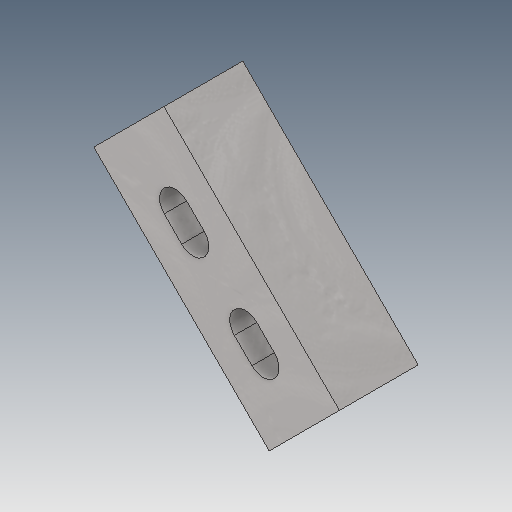
# Autodesk Inventor part: Conduit-brace
Saved by Autodesk Inventor 2017 (Build 210142000, 142)
## iProperties
Created: 2018-08-09
Part Number: Conduit-brace
Material: Generic
Document SubType Name: Modeling
Designer: Kathryn Rosie
Density: 1 g/cm^3
Appearance: Weld - Steel Mild
Author: Kathryn Rosie
Autodesk Inventor part; units mm, degrees
ref_plane "YZ Plane" through (0, 0, 0) normal (1, 0, 0) x (0, 1, 0)
ref_plane "XZ Plane" through (0, 0, 0) normal (0, 1, 0) x (-1, 0, 0)
ref_plane "XY Plane" through (0, 0, 0) normal (0, 0, 1) x (1, 0, 0)
sketch "Sketch1" plane through (0, 0, 0) normal (0, 0, 1) x (1, 0, 0)
  line L0 (7.0711, 21.2132) -> (20.3934, 34.5355)
  line L1 (61, 1) -> (41.6066, 20.3934)
  line L2 (61, 1) -> (725, 1)
  line L3 (725, 1) -> (725, 26)
  line L4 (725, 26) -> (720, 31)
  line L5 (720, 31) -> (437.7615, 31)
  arc A0 (434.226, 32.4645) -> (437.7615, 31) centre (437.7615, 36) ccw
  line L6 (434.226, 32.4645) -> (32.4645, 434.226)
  arc A1 (31, 437.7615) -> (32.4645, 434.226) centre (36, 437.7615) ccw
  line L7 (31, 437.7615) -> (31, 720)
  line L8 (31, 720) -> (26, 725)
  line L9 (26, 725) -> (1, 725)
  line L10 (1, 725) -> (1, 61)
  line L11 (20.3934, 41.6066) -> (1, 61)
  arc A2 (20.3934, 34.5355) -> (20.3934, 41.6066) centre (16.8579, 38.0711) ccw
  line L12 (7.0711, 21.2132) -> (20.3934, 34.5355)
  line L13 (21.2132, 7.0711) -> (7.0711, 21.2132)
  line L14 (34.5355, 20.3934) -> (21.2132, 7.0711)
  arc A3 (41.6066, 20.3934) -> (34.5355, 20.3934) centre (38.0711, 16.8579) ccw
  circle A4 centre (15, 600) radius 3.2
  circle A5 centre (200, 15) radius 3.2
  circle A6 centre (600, 15) radius 3.2
  line L15 (252.9319, 164.2611) -> (377.6575, 39.5355)
  arc A7 (374.1219, 31) -> (377.6575, 39.5355) centre (374.1219, 36) ccw
  line L16 (374.1219, 31) -> (82.5685, 31)
  arc A8 (79.033, 32.4645) -> (82.5685, 31) centre (82.5685, 36) ccw
  line L17 (79.033, 32.4645) -> (32.4645, 79.033)
  arc A9 (31, 82.5685) -> (32.4645, 79.033) centre (36, 82.5685) ccw
  line L18 (31, 82.5685) -> (31, 374.1219)
  arc A10 (39.5355, 377.6575) -> (31, 374.1219) centre (36, 374.1219) ccw
  line L19 (39.5355, 377.6575) -> (164.2611, 252.9319)
  arc A11 (162.7002, 244.8028) -> (164.2611, 252.9319) centre (160.7256, 249.3963) ccw
  arc A12 (162.7002, 244.8028) -> (244.8028, 162.7002) centre (187.3833, 187.3833) ccw
  arc A13 (252.9319, 164.2611) -> (244.8028, 162.7002) centre (249.3963, 160.7256) ccw
  circle A14 centre (15, 200) radius 3.2
  line L20 (-61, -1) -> (-41.6066, -20.3934)
  line L21 (-61, -1) -> (-725, -1)
  line L22 (-725, -1) -> (-725, -26)
  line L23 (-725, -26) -> (-720, -31)
  line L24 (-720, -31) -> (-437.7615, -31)
  arc A15 (-434.226, -32.4645) -> (-437.7615, -31) centre (-437.7615, -36) ccw
  line L25 (-434.226, -32.4645) -> (-32.4645, -434.226)
  arc A16 (-31, -437.7615) -> (-32.4645, -434.226) centre (-36, -437.7615) ccw
  line L26 (-31, -437.7615) -> (-31, -720)
  line L27 (-31, -720) -> (-26, -725)
  line L28 (-26, -725) -> (-1, -725)
  line L29 (-1, -725) -> (-1, -61)
  line L30 (-20.3934, -41.6066) -> (-1, -61)
  arc A17 (-20.3934, -34.5355) -> (-20.3934, -41.6066) centre (-16.8579, -38.0711) ccw
  line L31 (-7.0711, -21.2132) -> (-20.3934, -34.5355)
  line L32 (-21.2132, -7.0711) -> (-7.0711, -21.2132)
  line L33 (-34.5355, -20.3934) -> (-21.2132, -7.0711)
  arc A18 (-41.6066, -20.3934) -> (-34.5355, -20.3934) centre (-38.0711, -16.8579) ccw
  circle A19 centre (-15, -600) radius 3.2
  circle A20 centre (-200, -15) radius 3.2
  circle A21 centre (-600, -15) radius 3.2
  line L34 (-252.9319, -164.2611) -> (-377.6575, -39.5355)
  arc A22 (-374.1219, -31) -> (-377.6575, -39.5355) centre (-374.1219, -36) ccw
  line L35 (-374.1219, -31) -> (-82.5685, -31)
  arc A23 (-79.033, -32.4645) -> (-82.5685, -31) centre (-82.5685, -36) ccw
  line L36 (-79.033, -32.4645) -> (-32.4645, -79.033)
  arc A24 (-31, -82.5685) -> (-32.4645, -79.033) centre (-36, -82.5685) ccw
  line L37 (-31, -82.5685) -> (-31, -374.1219)
  arc A25 (-39.5355, -377.6575) -> (-31, -374.1219) centre (-36, -374.1219) ccw
  line L38 (-39.5355, -377.6575) -> (-164.2611, -252.9319)
  arc A26 (-162.7002, -244.8028) -> (-164.2611, -252.9319) centre (-160.7256, -249.3963) ccw
  arc A27 (-162.7002, -244.8028) -> (-244.8028, -162.7002) centre (-187.3833, -187.3833) ccw
  arc A28 (-252.9319, -164.2611) -> (-244.8028, -162.7002) centre (-249.3963, -160.7256) ccw
  circle A29 centre (-15, -200) radius 3.2
  line L39 (-1, 61) -> (-20.3934, 41.6066)
  line L40 (-1, 61) -> (-1, 725)
  line L41 (-1, 725) -> (-26, 725)
  line L42 (-26, 725) -> (-31, 720)
  line L43 (-31, 720) -> (-31, 437.7615)
  arc A30 (-32.4645, 434.226) -> (-31, 437.7615) centre (-36, 437.7615) ccw
  line L44 (-32.4645, 434.226) -> (-434.226, 32.4645)
  arc A31 (-437.7615, 31) -> (-434.226, 32.4645) centre (-437.7615, 36) ccw
  line L45 (-437.7615, 31) -> (-720, 31)
  line L46 (-720, 31) -> (-725, 26)
  line L47 (-725, 26) -> (-725, 1)
  line L48 (-725, 1) -> (-61, 1)
  line L49 (-41.6066, 20.3934) -> (-61, 1)
  arc A32 (-34.5355, 20.3934) -> (-41.6066, 20.3934) centre (-38.0711, 16.8579) ccw
  line L50 (-21.2132, 7.0711) -> (-34.5355, 20.3934)
  line L51 (-7.0711, 21.2132) -> (-21.2132, 7.0711)
  line L52 (-20.3934, 34.5355) -> (-7.0711, 21.2132)
  arc A33 (-20.3934, 41.6066) -> (-20.3934, 34.5355) centre (-16.8579, 38.0711) ccw
  circle A34 centre (-600, 15) radius 3.2
  circle A35 centre (-15, 200) radius 3.2
  circle A36 centre (-15, 600) radius 3.2
  line L53 (-164.2611, 252.9319) -> (-39.5355, 377.6575)
  arc A37 (-31, 374.1219) -> (-39.5355, 377.6575) centre (-36, 374.1219) ccw
  line L54 (-31, 374.1219) -> (-31, 82.5685)
  arc A38 (-32.4645, 79.033) -> (-31, 82.5685) centre (-36, 82.5685) ccw
  line L55 (-32.4645, 79.033) -> (-79.033, 32.4645)
  arc A39 (-82.5685, 31) -> (-79.033, 32.4645) centre (-82.5685, 36) ccw
  line L56 (-82.5685, 31) -> (-374.1219, 31)
  arc A40 (-377.6575, 39.5355) -> (-374.1219, 31) centre (-374.1219, 36) ccw
  line L57 (-377.6575, 39.5355) -> (-252.9319, 164.2611)
  arc A41 (-244.8028, 162.7002) -> (-252.9319, 164.2611) centre (-249.3963, 160.7256) ccw
  arc A42 (-244.8028, 162.7002) -> (-162.7002, 244.8028) centre (-187.3833, 187.3833) ccw
  arc A43 (-164.2611, 252.9319) -> (-162.7002, 244.8028) centre (-160.7256, 249.3963) ccw
  circle A44 centre (-200, 15) radius 3.2
  line L58 (1, -61) -> (20.3934, -41.6066)
  line L59 (1, -61) -> (1, -725)
  line L60 (1, -725) -> (26, -725)
  line L61 (26, -725) -> (31, -720)
  line L62 (31, -720) -> (31, -437.7615)
  arc A45 (32.4645, -434.226) -> (31, -437.7615) centre (36, -437.7615) ccw
  line L63 (32.4645, -434.226) -> (434.226, -32.4645)
  arc A46 (437.7615, -31) -> (434.226, -32.4645) centre (437.7615, -36) ccw
  line L64 (437.7615, -31) -> (720, -31)
  line L65 (720, -31) -> (725, -26)
  line L66 (725, -26) -> (725, -1)
  line L67 (725, -1) -> (61, -1)
  line L68 (41.6066, -20.3934) -> (61, -1)
  arc A47 (34.5355, -20.3934) -> (41.6066, -20.3934) centre (38.0711, -16.8579) ccw
  line L69 (21.2132, -7.0711) -> (34.5355, -20.3934)
  line L70 (7.0711, -21.2132) -> (21.2132, -7.0711)
  line L71 (20.3934, -34.5355) -> (7.0711, -21.2132)
  arc A48 (20.3934, -41.6066) -> (20.3934, -34.5355) centre (16.8579, -38.0711) ccw
  circle A49 centre (600, -15) radius 3.2
  circle A50 centre (15, -200) radius 3.2
  circle A51 centre (15, -600) radius 3.2
  line L72 (164.2611, -252.9319) -> (39.5355, -377.6575)
  arc A52 (31, -374.1219) -> (39.5355, -377.6575) centre (36, -374.1219) ccw
  line L73 (31, -374.1219) -> (31, -82.5685)
  arc A53 (32.4645, -79.033) -> (31, -82.5685) centre (36, -82.5685) ccw
  line L74 (32.4645, -79.033) -> (79.033, -32.4645)
  arc A54 (82.5685, -31) -> (79.033, -32.4645) centre (82.5685, -36) ccw
  line L75 (82.5685, -31) -> (374.1219, -31)
  arc A55 (377.6575, -39.5355) -> (374.1219, -31) centre (374.1219, -36) ccw
  line L76 (377.6575, -39.5355) -> (252.9319, -164.2611)
  arc A56 (244.8028, -162.7002) -> (252.9319, -164.2611) centre (249.3963, -160.7256) ccw
  arc A57 (244.8028, -162.7002) -> (162.7002, -244.8028) centre (187.3833, -187.3833) ccw
  arc A58 (164.2611, -252.9319) -> (162.7002, -244.8028) centre (160.7256, -249.3963) ccw
  circle A59 centre (200, -15) radius 3.2
  line L77 (-8.1812, 19.7495) -> (8.1812, 19.7495)
  line L78 (19.7495, 8.1812) -> (8.1812, 19.7495)
  line L79 (19.7495, 8.1812) -> (19.7495, -8.1812)
  line L80 (13.9654, -13.9654) -> (19.7495, -8.1812)
  line L81 (5.6569, -5.6569) -> (13.9654, -13.9654)
  arc A60 (5.6569, -5.6569) -> (-5.6569, 5.6569) centre (0, 0) ccw
  line L82 (-13.9654, 13.9654) -> (-5.6569, 5.6569)
  line L83 (-8.1812, 19.7495) -> (-13.9654, 13.9654)
  line L84 (8.1812, -19.7495) -> (-8.1812, -19.7495)
  line L85 (-19.7495, -8.1812) -> (-8.1812, -19.7495)
  line L86 (-19.7495, -8.1812) -> (-19.7495, 8.1812)
  line L87 (-13.9654, 13.9654) -> (-19.7495, 8.1812)
  line L88 (-5.6569, 5.6569) -> (-13.9654, 13.9654)
  arc A61 (-5.6569, 5.6569) -> (5.6569, -5.6569) centre (0, 0) ccw
  line L89 (13.9654, -13.9654) -> (5.6569, -5.6569)
  line L90 (8.1812, -19.7495) -> (13.9654, -13.9654)
  line L91 (-4.0659, 18.208) -> (-18.208, 4.0659)
  line L92 (-18.208, 4.0659) -> (-53.5633, 39.4212)
  line L93 (-18.208, 4.0659) -> (31.792, 4.0659) construction
  line L94 (-4.0659, 18.208) -> (-39.4212, 53.5633)
  line L95 (-45.1904, 45.1904) -> (-11.1369, 11.1369) construction
  line L96 (-19.4454, 19.4454) -> (-22.981, 22.981) construction
  line L97 (-17.1827, 21.7082) -> (-20.7182, 25.2437)
  line L98 (-25.2437, 20.7182) -> (-21.7082, 17.1827)
  arc A62 (-21.7082, 17.1827) -> (-17.1827, 21.7082) centre (-19.4454, 19.4454) ccw
  arc A63 (-20.7182, 25.2437) -> (-25.2437, 20.7182) centre (-22.981, 22.981) ccw
  line L99 (-33.5876, 33.5876) -> (-37.1231, 37.1231) construction
  line L100 (-31.3248, 35.8503) -> (-34.8604, 39.3858)
  line L101 (-39.3858, 34.8604) -> (-35.8503, 31.3248)
  arc A64 (-35.8503, 31.3248) -> (-31.3248, 35.8503) centre (-33.5876, 33.5876) ccw
  arc A65 (-34.8604, 39.3858) -> (-39.3858, 34.8604) centre (-37.1231, 37.1231) ccw
  line L102 (-53.5633, 39.4212) -> (-39.4212, 53.5633)
  point P0 (0, 0)
  point P1 (-21.2132, 21.2132)
  point P2 (-35.3553, 35.3553)
extrude "Extrusion2" add sketch "Sketch1" along normal blind 15.875 contours L52 L51 L50 L92 L102 L94 | L94 L77 L83 L87 L86 L92 L51 | L94 L91 L82 L83 L77 | L86 L87 L82 L91 L92
body "Solid2"
